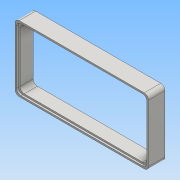
# Autodesk Inventor part: Box2_walls
Saved by Autodesk Inventor 2016 (Build 200138000, 138)
## iProperties
Created: 2015-09-13
Part Number: Box2_walls
Material: PPS Plastic
Document SubType Name: Modeling
Designer: Openlab
Density: 1.637 g/cm^3
Appearance: Smooth - White
Author: Openlab
Autodesk Inventor part; units mm, degrees
ref_plane "YZ Plane" through (0, 0, 0) normal (1, 0, 0) x (0, 1, 0)
ref_plane "XZ Plane" through (0, 0, 0) normal (0, 1, 0) x (-1, 0, 0)
ref_plane "XY Plane" through (0, 0, 0) normal (0, 0, 1) x (1, 0, 0)
sketch "Sketch1" plane through (0, 0, 0) normal (0, 1, 0) x (-1, 0, 0)
  line L0 (-70, 35) -> (70, 35)
  line L1 (75, 30) -> (75, -30)
  line L2 (70, -35) -> (-70, -35)
  line L3 (-75, -30) -> (-75, 30)
  line L4 (-75, 35) -> (75, -35) construction
  line L5 (75, 35) -> (-75, -35) construction
  arc A0 (75, 30) -> (70, 35) centre (70, 30) ccw
  arc A1 (70, -35) -> (75, -30) centre (70, -30) ccw
  arc A2 (-70, 35) -> (-75, 30) centre (-70, 30) ccw
  arc A3 (-75, -30) -> (-70, -35) centre (-70, -30) ccw
  line L6 (-72, 37) -> (72, 37)
  line L7 (77, 32) -> (77, -32)
  line L8 (72, -37) -> (-72, -37)
  line L9 (-77, -32) -> (-77, 32)
  line L10 (-77, 37) -> (77, -37) construction
  line L11 (77, 37) -> (-77, -37) construction
  arc A4 (77, 32) -> (72, 37) centre (72, 32) ccw
  arc A5 (72, -37) -> (77, -32) centre (72, -32) ccw
  arc A6 (-77, -32) -> (-72, -37) centre (-72, -32) ccw
  arc A7 (-72, 37) -> (-77, 32) centre (-72, 32) ccw
  line L12 (74, 39) -> (-74, 39)
  line L13 (-79, 34) -> (-79, -34)
  line L14 (-74, -39) -> (74, -39)
  line L15 (79, -34) -> (79, 34)
  line L16 (79, 39) -> (-79, -39) construction
  line L17 (-79, 39) -> (79, -39) construction
  arc A8 (79, 34) -> (74, 39) centre (74, 34) ccw
  arc A9 (-74, 39) -> (-79, 34) centre (-74, 34) ccw
  arc A10 (-79, -34) -> (-74, -39) centre (-74, -34) ccw
  arc A11 (74, -39) -> (79, -34) centre (74, -34) ccw
  point P0 (0, 0)
  dimension "d0" = 150
  dimension "d1" = 70
  dimension "d2" = 5
  dimension "d6" = 2
  dimension "d7" = 2
  dimension "d8" = 5
  dimension "d9" = 4
  dimension "d10" = 4
  dimension "d11" = 5
  constraints: 36 end point, 24 point on circle, 24 point on line, 24 tangent, 12 centre point, 9 equal radius, 6 midpoint, 6 parallel, 3 horizontal, 3 perpendicular
  measures "d0" distance of L4.end L5.end
  measures "d1" distance of L5.start L4.end
  measures "d2" radius of A0
  measures "d6" distance between parallel lines of L8 L2
  measures "d7" distance between parallel lines of L7 L1
  measures "d8" radius of A4
  measures "d9" distance between parallel lines of L15 L1
  measures "d10" distance between parallel lines of L14 L2
  measures "d11" radius of A8
extrude "Extrusion1" add sketch "Sketch1" along normal mid plane 15.5 contours L6 A4 L7 A5 L8 A6 L9 A7
extrude "Extrusion2" add sketch "Sketch1" along normal mid plane 19.5 contours A8 L15 A11 L14 A10 L13 A9 L12
body "Solid1"
